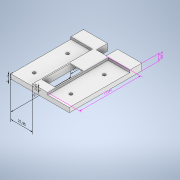
# Autodesk Inventor part: floor-4
Saved by Autodesk Inventor 2020 (Build 240168000, 168)
## iProperties
Created: 2019-10-25
Part Number: floor-4
Material: ABS Plastic
Document SubType Name: Modeling
Designer: sl65b
Density: 1.06 g/cm^3
Appearance: Smooth - White
Mass: 43.4032 g
Surface Area: 160.957 cm^2
Volume: 40.9464 cm^3
Author: sl65b
Autodesk Inventor part; units mm, degrees
ref_plane "YZ Plane" through (0, 0, 0) normal (1, 0, 0) x (0, 1, 0)
ref_plane "XZ Plane" through (0, 0, 0) normal (0, 1, 0) x (-1, 0, 0)
ref_plane "XY Plane" through (0, 0, 0) normal (0, 0, 1) x (1, 0, 0)
sketch "Sketch1" plane through (0, 0, 0) normal (0, 1, 0) x (-1, 0, 0)
  line L0 (-35, 36.5) -> (35, 36.5)
  line L1 (35, 36.5) -> (35, -36.5)
  line L2 (35, -36.5) -> (-35, -36.5)
  line L3 (-35, -36.5) -> (-35, 36.5)
  line L4 (-35, 36.5) -> (35, -36.5) construction
  line L5 (35, 36.5) -> (-35, -36.5) construction
  line L6 (-35, -36.5) -> (-35, -50.5)
  line L7 (-35, -50.5) -> (-6, -50.5)
  line L8 (6.0499, -50.5) -> (35, -50.5)
  line L9 (35, -50.5) -> (35, -36.5)
  line L10 (6.0499, -36.5) -> (6.0499, -43.5)
  line L11 (6.0499, -43.5) -> (-6, -43.5)
  line L12 (-6, -43.5) -> (-6, -36.5)
  line L13 (-6, -50.5) -> (-6, -43.5)
  line L14 (6.0499, -50.5) -> (6.0499, -43.5)
  point P0 (0, 0)
  dimension "d0" = 70
  dimension "d1" = 73
  dimension "d2" = 14
  dimension "d3" = 29
  dimension "d4" = 7
  dimension "d5" = 87
  dimension "d61" = 7
  dimension "d64" = 12.0499
  constraints: 30 end point, 3 equal length, 3 perpendicular, 2 midpoint, 2 point on line, 2 vertical, 1 horizontal
  measures "d0" distance of L0.start L0.end
  measures "d1" distance of L2.end L0.start
  measures "d2" distance of L2.end L6.end
  measures "d3" distance of L6.end L7.end
  measures "d4" distance of L10.start L10.end
  measures "d5" distance between parallel lines of L0 L8
  measures "d61" distance of L11.end L12.end
  measures "d64" distance between parallel lines of L12 L10
sketch "Sketch2" plane through (0, 0, 0) normal (0, 1, 0) x (-1, 0, 0)
  point P0 (0, 0)
extrude "Extrusion1" add sketch "Sketch1" along normal blind 8 contours L0 L1 L2 L3 | L2 L12 L13 L7 L6 | L9 L8 L14 L10 L2
sketch "Sketch3" plane through (0, 8, 0) normal (0, 1, 0) x (1, 0, 0)
  line L0 (9, 36) -> (9, -36.5)
  line L1 (35, -36.5) -> (35, 36)
  line L2 (9, 36) -> (35, 36)
  line L3 (6, 50.5) -> (6, 36.5) projected
  line L4 (-9.0499, -36.5) -> (-9.0499, 35.5)
  line L5 (-9.0499, 35.5) -> (-35, 35.5)
  line L6 (-35, 35.5) -> (-35, -36.5)
  line L7 (-35, -36.5) -> (-9.0499, -36.5)
  line L8 (-6.0499, 36.5) -> (-6.0499, 50.5) projected
  line L9 (9, -36.5) -> (35, -36.5)
  point P0 (0, 0)
  point P1 (6, 43.5)
  point P2 (-6.0499, 43.5)
  dimension "d8" = 3
  dimension "d9" = 3
  constraints: 16 end point, 2 vertical, 1 horizontal, 1 perpendicular
  measures "d8" distance between parallel lines of L0 L3
  measures "d9" distance between parallel lines of L8 L4
extrude "Extrusion2" cut sketch "Sketch3" against normal blind 2.61
sketch "Sketch4" plane through (0, 0, 0) normal (0, -1, 0) x (1, 0, 0)
  line L0 (-35, 36.5) -> (35, 36.5) projected
  line L1 (-29.525, 36.5) -> (-29.525, -42.6114)
  line L2 (-35, -50.5) -> (-35, 36.5) projected
  line L3 (29.525, 36.5) -> (29.525, -43.7753)
  line L4 (35, 36.5) -> (35, -50.5) projected
  line L5 (-14.525, 36.5) -> (-14.525, -22.6051)
  line L6 (14.5, 36.5) -> (14.5, -47.1695)
  line L7 (-22.025, 36.5) -> (-22.025, -33.1573)
  line L8 (-22.025, 36.5) -> (-22.025, 23.3)
  circle A0 centre (-22.025, 21.55) radius 1.75
  line L9 (-9.0499, 36.5) -> (9, 36.5) projected
  line L10 (22, 36.5) -> (22, -38.3698)
  line L11 (22, 36.5) -> (22, 23.3)
  circle A1 centre (22, 21.55) radius 1.75
  circle A2 centre (22, -18.45) radius 1.75
  circle A3 centre (-22.025, -18.45) radius 1.75
  point P0 (0, 0)
  point P1 (-35, -56.5)
  point P2 (22.1782, -20.1909)
  point P3 (-23.772, -18.5519)
  dimension "d40" = 3.5
  dimension "d45" = 3.5
  dimension "d46" = 3.5
  dimension "d47" = 36.5
  dimension "d48" = 3.5
  dimension "d31" = 5.475
  dimension "d32" = 5.475
  dimension "d33" = 15
  dimension "d38" = 7.5
  dimension "d39" = 13.2
  dimension "d43" = 7.5
  dimension "d44" = 13.2
  dimension "d49" = 40
  dimension "d57" = 14.525
  constraints: 16 end point, 7 point on line, 6 vertical, 2 vertical alignment, 16 other
  measures "d31" distance between parallel lines of L2 L1
  measures "d32" distance between parallel lines of L3 L4
  measures "d33" distance between parallel lines of L1 L5
  measures "d38" distance between parallel lines of L5 L7
  measures "d39" distance of L7.start L8.end
  measures "d43" distance between parallel lines of L6 L10
  measures "d44" distance of L10.start L11.end
  measures "d49" distance of point (-22.025, -18.45) point (-22.025, 21.55)
  measures "d57" distance from line of point (0, 0) L5
hole "Hole1" at (22, 0, 21.55) at (22, 0, -18.45) at (-22.025, 0, 21.55) at (-22.025, 0, -18.45) direction (0, 1, 0) diameter 3.5 depth 15.664 counterbore diameter 10 counterbore depth 2
sketch "Sketch5" plane through (6, 0, -36.5) normal (0, 0, -1) x (-1, 0, 0)
  line L0 (41, 0) -> (-29, 0) projected
  line L1 (0, 0) -> (15.0499, 0)
  line L2 (15.0499, 0) -> (15.0499, 8)
  line L3 (15.0499, 8) -> (0, 8)
  line L4 (0, 8) -> (0, 0)
  point P0 (6, 0)
  constraints: 8 end point, 2 parallel, 1 horizontal, 1 perpendicular, 1 point on line
extrude "Extrusion3" add sketch "Sketch5" along normal blind 0.5
sketch "Sketch10" plane through (0, 0, 0) normal (0, -1, 0) x (1, 0, 0)
  line L0 (-7.6499, -30) -> (-7.6499, 26.5)
  line L1 (-7.6499, 26.5) -> (7.6, 26.5)
  line L2 (7.6, 26.5) -> (7.6, -30)
  line L3 (7.6, -30) -> (-7.6499, -30)
  line L4 (6, -37) -> (-6.0499, -37) projected
  line L5 (-35, 36.5) -> (35, 36.5) projected
  line L6 (9, 36.5) -> (9, -36) projected
  line L7 (-9.0499, -35.5) -> (-9.0499, 36.5) projected
  point P0 (0, 0)
  dimension "d72" = 7
  dimension "d73" = 10
  dimension "d74" = 1.4
  dimension "d75" = 1.4
  constraints: 8 end point, 3 perpendicular, 1 vertical
  measures "d72" distance between parallel lines of L4 L3
  measures "d73" distance between parallel lines of L5 L1
  measures "d74" distance between parallel lines of L6 L2
  measures "d75" distance between parallel lines of L7 L0
extrude "Extrusion4" cut sketch "Sketch10" against normal blind 7
sketch "Sketch12" plane through (6, 0, -37) normal (0, 0, -1) x (-1, 0, 0)
  line L0 (12.0499, 0) -> (12.0499, 8) projected
  line L1 (0, 0) -> (0, 8) projected
  circle A0 centre (3.025, 4) radius 1.5
  circle A1 centre (9.025, 4) radius 1.5
  line L2 (6.025, 1.0105) -> (6.025, 8)
  line L3 (12.0499, 8) -> (0, 8) projected
  point P0 (6, 0)
  dimension "d78" = 12.0499
  dimension "d79" = 3
  dimension "d80" = 3
  dimension "d82" = 3
  dimension "d83" = 3
  dimension "d84" = 2.5
  constraints: 2 centre point, 2 end point, 1 vertical
  measures "d78" distance between parallel lines of L0 L1
  measures "d79" diameter of A0
  measures "d80" diameter of A1
  measures "d82" distance from line of L2 A0.centre
  measures "d83" distance from line of L2 A1.centre
  measures "d84" distance edge to line of A0 L3
hole "Hole2" at (2.975, 4, -37) at (-3.025, 4, -37) direction (0, 0, 1) diameter 3 depth 10.5 tip angle 118
sketch "Sketch13" plane through (0, 8, 0) normal (0, 1, 0) x (1, 0, 0)
  line L0 (-7.6499, -26.5) -> (7.6, -26.5) projected
  line L1 (-7.7014, -26.5) -> (7.6, -26.5)
  line L2 (7.6, -26.5) -> (7.6, 7.4212)
  line L3 (7.6, -26.5) -> (7.6, 30) projected
  line L4 (-7.6499, 7.4212) -> (-7.6499, -26.5)
  line L5 (-7.6499, 7.4212) -> (7.6, 7.4212)
  point P0 (0, 0)
  point P1 (8.2986, -26.5)
  constraints: 8 end point, 4 point on line, 1 parallel, 1 perpendicular
extrude "Extrusion5" cut sketch "Sketch13" against normal blind 10
body "Solid1"
